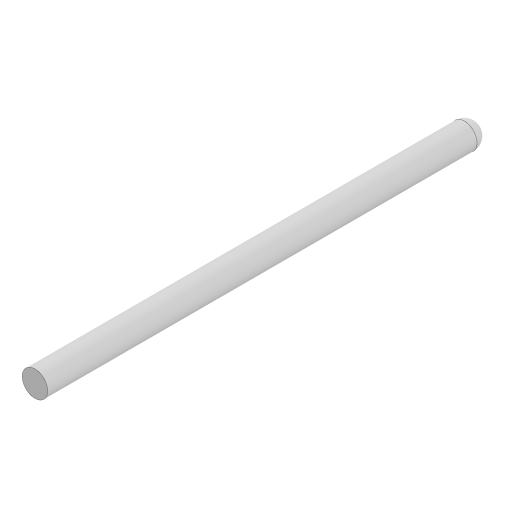
# Autodesk Inventor part: stylus_nib
Saved by Autodesk Inventor 2023 (Build 270158000, 158)
## iProperties
Created: 2023-03-22
Part Number: stylus_nib
Material: Generic
Document SubType Name: Modeling
Designer: James
Density: 1 g/cm^3
Appearance: Default
Author: James
Autodesk Inventor part; units mm, degrees
ref_plane "YZ Plane" through (0, 0, 0) normal (1, 0, 0) x (0, 1, 0)
ref_plane "XZ Plane" through (0, 0, 0) normal (0, 1, 0) x (-1, 0, 0)
ref_plane "XY Plane" through (0, 0, 0) normal (0, 0, 1) x (1, 0, 0)
sketch "Sketch1" plane through (0, 0, 0) normal (0, 1, 0) x (-1, 0, 0)
  line L0 (0, 0) -> (0.75, 0)
  line L1 (0.75, 0) -> (0.75, -25.25)
  line L2 (0, -26) -> (0, 0)
  arc A0 (0, -26) -> (0.75, -25.25) centre (0, -25.25) ccw
  dimension "d4" = 26
  dimension "d5" = 0.75
  constraints: 6 end point, 2 point on circle, 1 centre point, 1 horizontal, 1 line through centre, 1 parallel, 1 perpendicular, 1 tangent
  measures "d4" distance of L2.start L0.start
  measures "d5" distance between parallel lines of L2 L1
revolve "Revolution1" add sketch "Sketch1" angle 360 about axis through (0, 0, -26) along (0, 0, 1)
body "Solid1"
